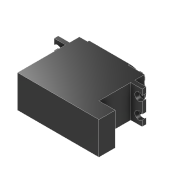
# Autodesk Inventor part: Motorv2
Saved by Autodesk Inventor 2022 (Build 260153000, 153)
## iProperties
Created: 2022-02-23
Part Number: Motorv2
Material: Generic
Document SubType Name: Modeling
Designer: piers
Density: 1 g/cm^3
Appearance: Glossy - Black
Author: piers
Autodesk Inventor part; units mm, degrees
ref_plane "YZ Plane" through (0, 0, 0) normal (1, 0, 0) x (0, 1, 0)
ref_plane "XZ Plane" through (0, 0, 0) normal (0, 1, 0) x (-1, 0, 0)
sketch "Sketch1" plane through (0, 0, 0) normal (0, 0, 1) x (1, 0, 0)
  line L0 (7, 0) -> (47, 0)
  line L1 (47, 20) -> (7, 20)
  line L2 (7, 20) -> (7, 0)
  line L3 (47, 20) -> (47, 0)
  point P0 (0, 0)
  constraints: 8 end point, 2 perpendicular, 1 horizontal, 1 parallel
extrude "Extrusion1" add sketch "Sketch1" along normal blind 28 and the other way blind 10
sketch "Sketch2" plane through (0, 0, -10) normal (0, 0, -1) x (-1, 0, 0)
  line L0 (-7, 20) -> (-47, 20) projected
  line L1 (-47, 20) -> (-47, 10)
  line L2 (-47, 20) -> (-47, 0) projected
  line L3 (-47, 10) -> (-37, 10)
  circle A0 centre (-37, 10) radius 2.5
  point P0 (0, 0)
  dimension "d10" = 10
  dimension "d11" = 10
  dimension "d12" = 5
  constraints: 4 end point, 1 centre point, 1 coincident, 1 midpoint, 1 perpendicular
  measures "d10" distance of L0.end L1.end
  measures "d11" distance of L1.end L3.end
  measures "d12" diameter of A0
extrude "Extrusion3" add sketch "Sketch2" along normal blind 8
sketch "Sketch3" plane through (0, 0, -10) normal (0, 0, -1) x (-1, 0, 0)
  circle A0 centre (-37, 10) radius 2.5 projected
  circle A1 centre (-37, 10) radius 10
  line L0 (-47, 20) -> (-7, 20) projected
  line L1 (-7, 20) -> (0, 20) projected
  line L2 (-7, 20) -> (-12, 20)
  line L3 (-7, 20) -> (-47, 20) projected
  line L4 (-12, 20) -> (-12, 0)
  line L5 (-7, 0) -> (-47, 0) projected
  line L6 (-47, 0) -> (-7, 0) projected
  point P0 (0, 0)
  point P1 (-37, 0)
  point P2 (-37, 20)
  dimension "d15" = 5
  constraints: 4 end point, 1 centre point, 1 coincident, 1 collinear, 1 point on line, 1 tangent, 1 vertical
  measures "d15" distance of L0.end L2.end
extrude "Extrusion4" add sketch "Sketch3" along normal blind 1
ref_plane "Work Plane1" through (0, 0, -4) normal (0, 0, 1) x (1, 0, 0)
sketch "Sketch4" plane through (0, 0, -4) normal (0, 0, 1) x (1, 0, 0)
  line L0 (47, 0) -> (47, 20) projected
  line L1 (47, 20) -> (54, 20)
  line L2 (54, 0) -> (47, 0)
  line L3 (47, 20) -> (7, 20) projected
  line L4 (47, 0) -> (47, 20)
  line L5 (7, 20) -> (7, 0) projected
  line L6 (7, 0) -> (0, 0)
  line L7 (0, 20) -> (7, 20)
  line L8 (7, 10) -> (7, 15)
  line L9 (7, 15) -> (2, 15)
  arc A0 (0, 13.5) -> (0, 16.5) centre (2, 15) ccw
  line L10 (27, 10) -> (22.2315, 10)
  line L11 (47, 20) -> (47, 10) projected
  line L12 (47, 20) -> (27, 20)
  line L13 (27, 20) -> (27, 13.3752)
  arc A1 (0, 3.5) -> (0, 6.5) centre (2, 5) ccw
  arc A2 (54, 16.5) -> (54, 13.5) centre (52, 15) ccw
  arc A3 (54, 6.5) -> (54, 3.5) centre (52, 5) ccw
  line L14 (54, 20) -> (54, 16.5)
  line L15 (54, 13.5) -> (54, 6.5)
  line L16 (54, 3.5) -> (54, 0)
  line L17 (0, 0) -> (0, 3.5)
  line L18 (0, 6.5) -> (0, 13.5)
  line L19 (0, 16.5) -> (0, 20)
  dimension "d19" = 7
  dimension "d21" = 7
  dimension "d22" = 5
  dimension "d23" = 5
  dimension "d24" = 5
  dimension "d25" = 20
  constraints: 32 end point, 13 perpendicular, 8 point on circle, 4 centre point, 3 horizontal, 3 symmetric about line, 2 midpoint, 1 coincident, 1 point on line, 3 other
  measures "d19" distance of L0.end L1.end
  measures "d21" distance of L5.end L6.end
  measures "d22" distance of L8.start L8.end
  measures "d23" distance of L8.end L9.end
  measures "d24" diameter of A0
  measures "d25" distance of L0.end L12.end
extrude "Extrusion5" add sketch "Sketch4" along normal blind 2.5
sketch "Sketch5" plane through (0, 0, -11) normal (0, 0, -1) x (-1, 0, 0)
  circle A0 centre (-37, 10) radius 2.5 projected
  circle A1 centre (-37, 10) radius 2.5 projected
  circle A2 centre (-37, 10) radius 6.5
  point P0 (0, 0)
  dimension "d28" = 13
  constraints: 1 centre point, 1 coincident
  measures "d28" diameter of A2
extrude "Extrusion6" add sketch "Sketch5" along normal blind 2
sketch "Sketch6" plane through (47, 0, 28) normal (1, 0, 0) x (0, 0, -1)
  line L0 (29.5, 0) -> (0, 0) projected
  line L1 (0, 0) -> (10, 0)
  line L2 (10, 0) -> (10, 20)
  line L3 (0, 20) -> (29.5, 20) projected
  line L4 (0, 20) -> (10, 20)
  line L5 (0, 0) -> (0, 20) projected
  point P0 (28, 0)
  dimension "d31" = 10
  constraints: 6 end point, 2 perpendicular, 2 point on line
  measures "d31" distance of L0.end L1.end
extrude "Extrusion7" add sketch "Sketch6" along normal blind 10
body "Solid1"
